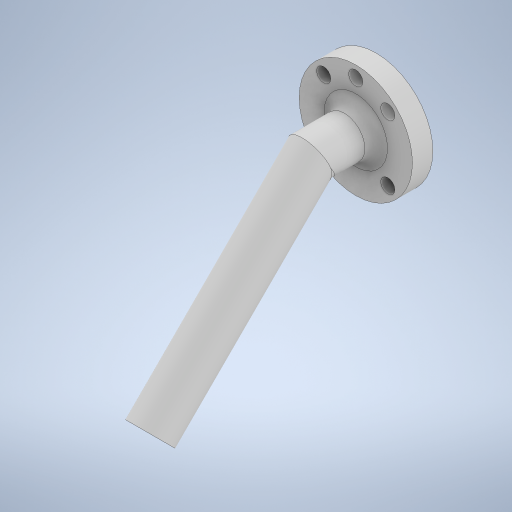
# Autodesk Inventor part: PenTool
Saved by Autodesk Inventor 2024.2 (Build 282272000, 272)
## iProperties
Created: 2024-02-26
Part Number: PenTool
Material: Generic
Document SubType Name: Sheet Metal
Designer: parmo
Density: 1 g/cm^3
Sheet Metal Rule: Default
Appearance: Default
Author: parmo
Autodesk Inventor part; units mm, degrees
ref_plane "YZ Plane" through (0, 0, 0) normal (1, 0, 0) x (0, 1, 0)
ref_plane "XZ Plane" through (0, 0, 0) normal (0, 1, 0) x (-1, 0, 0)
ref_plane "XY Plane" through (0, 0, 0) normal (0, 0, 1) x (1, 0, 0)
sketch "Sketch1" plane through (0, 0, 0) normal (0, 0, 1) x (1, 0, 0)
  circle A0 centre (0, 0) radius 12.5
  circle A1 centre (0, 0) radius 25
  circle A2 centre (0, 20) radius 3.125
  circle A3 centre (-14.1421, 14.1421) radius 3.125
  circle A4 centre (14.1421, 14.1421) radius 3.125
  circle A5 centre (-14.1421, -14.1421) radius 3.125
  circle A6 centre (14.1421, -14.1421) radius 3.125
  dimension "d1" = 25
  dimension "d2" = 50
  dimension "d3" = 6.25
  dimension "d5" = 6.25
  dimension "d7" = 6.25
  dimension "d10" = 6.25
  dimension "d11" = 6.25
  constraints: 7 centre point, 1 coincident
  measures "d1" diameter of A0
  measures "d2" diameter of A1
  measures "d3" diameter of A2
  measures "d5" diameter of A3
  measures "d7" diameter of A4
  measures "d10" diameter of A5
  measures "d11" diameter of A6
extrude "Extrusion1" add sketch "Sketch1" along normal blind 9 contours A0 | A1
sketch "Sketch4" plane through (0, 0, 0) normal (1, 0, 0) x (0, 1, 0)
  point P0 (0, 0)
sketch "Sketch5" plane through (0, 0, 0) normal (1, 0, 0) x (0, 1, 0)
  line L0 (0, 0) -> (0, 9)
  line L1 (0, 9) -> (0, 29)
  line L2 (0, 29) -> (-70.7107, 99.7107)
  line L3 (0, 29) -> (100, 29) construction
  dimension "d29" = 9
  dimension "d30" = 20
  dimension "d31" = 100
  dimension "d32" = 135
  constraints: 8 end point, 1 equal length, 1 horizontal, 1 point on line, 1 vertical
  measures "d29" distance of L0.start L0.end
  measures "d30" distance of L0.end L1.end
  measures "d31" distance of L1.end L2.end
  measures "d32" angle of L3 L2
sketch "Sketch6" plane through (0, 0, 9) normal (0, 0, 1) x (1, 0, 0)
  circle A0 centre (0, 0) radius 9
  dimension "d33" = 18
  constraints: 1 centre point, 1 coincident
  measures "d33" diameter of A0
sweep "Sweep1" add profiles "Sketch6" path "Sketch5"
sketch "Sketch8" plane through (0, -70.7107, 99.7107) normal (0, -0.7071068, 0.7071068) x (1, 0, 0)
  circle A0 centre (0, 0) radius 6.375
  point P0 (0, -20.5061)
  dimension "d36" = 12.75
  constraints: 1 centre point, 1 coincident
  measures "d36" diameter of A0
extrude "Extrusion3" cut sketch "Sketch8" against normal blind 100
fillet "Fillet2" radius 5 1 edges at (-9, 0, 9)
fillet "Fillet3" radius 5 1 edges at (0, -9, 25.2721)
equation "\"BendRadius\" = Thickness"
equation "\"BendReliefWidth\" = Thickness"
equation "\"BendReliefDepth\" = 0.5 * Thickness"
equation "\"CornerReliefSize\" = 4 * Thickness"
equation "\"MinimumRemnant\" = 2 * Thickness"
equation "\"TransitionRadius\" = BendRadius"
equation "\"JacobiRadiusSize\" = BendRadius"
equation "\"GapSize\" = Thickness"
equation "\"Thickness\" = 3.048"
body "Solid1"
